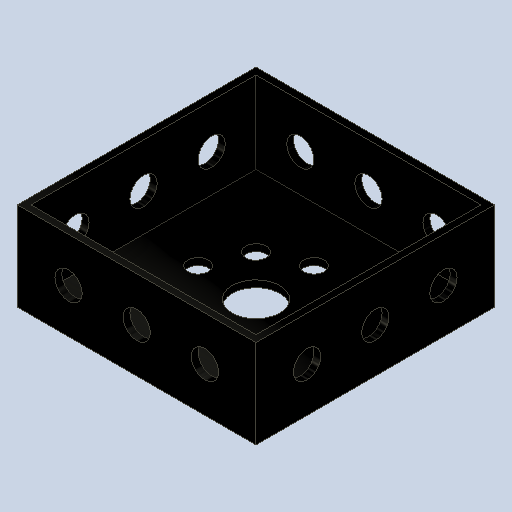
# Autodesk Inventor part: 01_Крепление_мотора
Saved by Autodesk Inventor 2022 (Build 260153000, 153)
## iProperties
Created: 2020-01-10
Part Number: 01_Крепление_мотора
Material: Сталь
Document SubType Name: Modeling
Designer: korsh
Density: 7.85 g/cm^3
Appearance: Оружейный металл
Mass: 20.4977 g
Surface Area: 56.1053 cm^2
Volume: 2.61117 cm^3
Author: korsh
Autodesk Inventor part; units mm, degrees
ref_plane "YZ Plane" through (0, 0, 0) normal (1, 0, 0) x (0, 1, 0)
ref_plane "XZ Plane" through (0, 0, 0) normal (0, 1, 0) x (-1, 0, 0)
ref_plane "XY Plane" through (0, 0, 0) normal (0, 0, 1) x (1, 0, 0)
sketch "Эскиз1" plane through (0, 0, 0) normal (0, 1, 0) x (-1, 0, 0)
  circle A0 centre (0, 0) radius 3.5
  circle A1 centre (0, -8.5) radius 1.5
  circle A2 centre (6.0104, -6.0104) radius 1.5
  circle A3 centre (8.5, 0) radius 1.5
  circle A4 centre (6.0104, 6.0104) radius 1.5
  circle A5 centre (0, 8.5) radius 1.5
  circle A6 centre (-6.0104, 6.0104) radius 1.5
  circle A7 centre (-8.5, 0) radius 1.5
  circle A8 centre (-6.0104, -6.0104) radius 1.5
  line L0 (17.5, 17.5) -> (-17.5, 17.5)
  line L1 (-17.5, 17.5) -> (-17.5, -17.5)
  line L2 (-17.5, -17.5) -> (17.5, -17.5)
  line L3 (17.5, -17.5) -> (17.5, 17.5)
  dimension "d0" = 7
  dimension "d1" = 3
  dimension "d2" = 8.5
  dimension "d5" = 360
  dimension "d7" = 35
  dimension "d8" = 17.5
  dimension "d9" = 35
  dimension "d10" = 17.5
  constraints: 9 centre point, 8 end point, 2 parallel, 1 coincident, 1 horizontal, 1 perpendicular, 17 other
  measures "d0" diameter of A0
  measures "d1" diameter of A1
  measures "d2" distance of point (0, 0) A1.centre
  measures "d7" distance of L0.start L0.end
  measures "d8" distance from line of point (0, 0) L3
  measures "d9" distance of L2.end L0.start
  measures "d10" distance from line of A0.centre L2
extrude "Выдавливание1" add sketch "Эскиз1" along normal blind 1
sketch "Эскиз2" plane through (0, 1, 0) normal (0, 1, 0) x (1, 0, 0)
  circle A0 centre (0, 0) radius 3.5 projected
  circle A1 centre (6.0104, 6.0104) radius 1.5 projected
  circle A2 centre (8.5, 0) radius 1.5 projected
  circle A3 centre (6.0104, -6.0104) radius 1.5 projected
  circle A4 centre (0, -8.5) radius 1.5 projected
  circle A5 centre (-6.0104, -6.0104) radius 1.5 projected
  circle A6 centre (-8.5, 0) radius 1.5 projected
  circle A7 centre (-6.0104, 6.0104) radius 1.5 projected
  circle A8 centre (0, 8.5) radius 1.5 projected
  line L0 (-17.5, -17.5) -> (17.5, -17.5) projected
  line L1 (17.5, -17.5) -> (17.5, 17.5) projected
  line L2 (17.5, 17.5) -> (-17.5, 17.5) projected
  line L3 (-17.5, 17.5) -> (-17.5, -17.5) projected
  line L4 (-16.5, -16.5) -> (16.5, -16.5)
  line L5 (16.5, -16.5) -> (16.5, 16.5)
  line L6 (16.5, 16.5) -> (-16.5, 16.5)
  line L7 (-16.5, 16.5) -> (-16.5, -16.5)
  dimension "d13" = 1
  dimension "d14" = 1
  dimension "d15" = 1
  dimension "d16" = 1
  constraints: 8 end point, 2 parallel, 1 horizontal, 1 perpendicular
  measures "d13" distance between parallel lines of L7 L3
  measures "d14" distance between parallel lines of L6 L2
  measures "d15" distance between parallel lines of L5 L1
  measures "d16" distance between parallel lines of L4 L0
extrude "Выдавливание2" add sketch "Эскиз2" along normal blind 12 contours L3 L2 L1 L0
sketch "Эскиз3" plane through (17.5, 0, 17.5) normal (1, 0, 0) x (0, 0, -1)
  circle A0 centre (17.5, 6.5) radius 2
  line L0 (0, 0) -> (0, 13) projected
  line L1 (35, 0) -> (35, 13) projected
  line L2 (0, 0) -> (35, 0) projected
  line L3 (0, 13) -> (35, 13) projected
  circle A1 centre (27.5, 6.5) radius 2
  circle A2 centre (7.5, 6.5) radius 2
  point P0 (17.5, 0)
  dimension "d19" = 4
  dimension "d20" = 35
  dimension "d21" = 17.5
  dimension "d22" = 13
  dimension "d23" = 6.5
  dimension "d24" = 4
  dimension "d25" = 10
  dimension "d26" = 4
  dimension "d27" = 10
  constraints: 3 centre point
  measures "d19" diameter of A0
  measures "d20" distance between parallel lines of L0 L1
  measures "d21" distance from line of A0.centre L1
  measures "d22" distance between parallel lines of L2 L3
  measures "d23" distance from line of A0.centre L3
  measures "d24" diameter of A1
  measures "d25" distance of A0.centre A1.centre
  measures "d26" diameter of A2
  measures "d27" distance of A2.centre A0.centre
extrude "Выдавливание3" cut sketch "Эскиз3" against normal blind 40 contours A0 | A1 | A2
sketch "Эскиз4" plane through (-17.5, 0, 17.5) normal (0, 0, 1) x (1, 0, 0)
  circle A0 centre (17.5, 6.5) radius 2
  line L0 (35, 0) -> (35, 13) projected
  line L1 (0, 0) -> (0, 13) projected
  line L2 (0, 0) -> (35, 0) projected
  line L3 (0, 13) -> (35, 13) projected
  circle A1 centre (27.5, 6.5) radius 2
  circle A2 centre (7.5, 6.5) radius 2
  point P0 (17.5, 0)
  dimension "d30" = 4
  dimension "d31" = 35
  dimension "d32" = 13
  dimension "d33" = 6.5
  dimension "d34" = 17.5
  dimension "d35" = 4
  dimension "d36" = 10
  dimension "d39" = 360
  constraints: 3 centre point, 5 other
  measures "d30" diameter of A0
  measures "d31" distance between parallel lines of L0 L1
  measures "d32" distance between parallel lines of L2 L3
  measures "d33" distance from line of L3 A0.centre
  measures "d34" distance from line of A0.centre L0
  measures "d35" diameter of A1
  measures "d36" distance of A0.centre A1.centre
extrude "Выдавливание4" cut sketch "Эскиз4" against normal blind 40 contours A0 | A1 | A2
equation "\"d8\" = 0.5 * d7"
equation "\"d9\" = d7"
equation "\"d10\" = 0.5 * d9"
equation "\"d14\" = d13"
equation "\"d15\" = d13"
equation "\"d16\" = d13"
equation "\"d21\" = 0.5 * d20"
equation "\"d23\" = 0.5 * d22"
equation "\"d33\" = 0.5 * d32"
equation "\"d34\" = 0.5 * d31"
